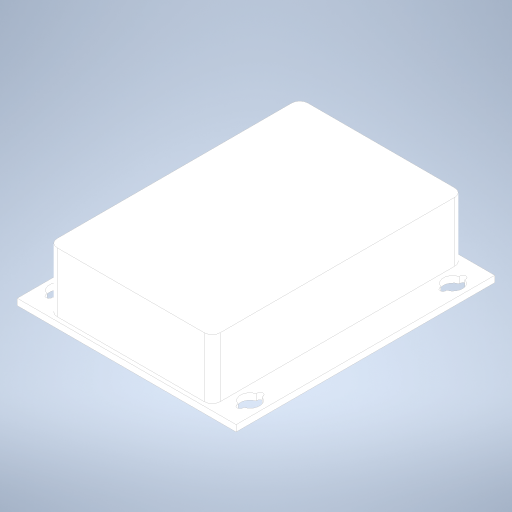
# Autodesk Inventor part: SUSTAINA-POWER-DISTRIBUTION-BOARD
Saved by Autodesk Inventor 2024.2 (Build 282272000, 272)
## iProperties
Created: 2024-01-24
Part Number: SUSTAINA-POWER-DISTRIBUTION-BOARD
Material: Acetal Resin, Black
Document SubType Name: Modeling
Designer: Masato Kubotera
Density: 1.425 g/cm^3
Appearance: Smooth - Black
Mass: 96.6275 g
Surface Area: 146.337 cm^2
Volume: 67.8088 cm^3
Author: Masato Kubotera
Autodesk Inventor part; units mm, degrees
ref_plane "YZ Plane" through (0, 0, 0) normal (1, 0, 0) x (0, 1, 0)
ref_plane "XZ Plane" through (0, 0, 0) normal (0, 1, 0) x (-1, 0, 0)
ref_plane "XY Plane" through (0, 0, 0) normal (0, 0, 1) x (1, 0, 0)
sketch "Sketch1" plane through (0, 0, 0) normal (0, 0, 1) x (1, 0, 0)
  line L0 (32.5, 27.5) -> (-32.5, 27.5)
  line L1 (-32.5, 27.5) -> (-32.5, -27.5)
  line L2 (-32.5, -27.5) -> (32.5, -27.5)
  line L3 (32.5, -27.5) -> (32.5, 27.5)
  line L4 (32.5, 27.5) -> (-32.5, -27.5) construction
  line L5 (-32.5, 27.5) -> (32.5, -27.5) construction
  line L6 (-25.5, 24) -> (25.5, 24) construction
  line L7 (25.5, 24) -> (25.5, -24) construction
  line L8 (25.5, -24) -> (-25.5, -24) construction
  line L9 (-25.5, -24) -> (-25.5, 24) construction
  line L10 (-25.5, 24) -> (25.5, -24) construction
  line L11 (25.5, 24) -> (-25.5, -24) construction
  line L12 (32.5, 0) -> (-32.5, 0) construction
  line L13 (0, 27.5) -> (0, -27.5) construction
  circle A0 centre (25.5, 24) radius 2.4
  circle A1 centre (-25.5, 24) radius 2.4
  circle A2 centre (25.5, -24) radius 2.4
  circle A3 centre (-25.5, -24) radius 2.4
  line L14 (25.5, 27.25) -> (25.5, 20.75) construction
  arc A4 (27.7895, 23.2801) -> (27.7895, 24.7199) centre (28, 24) ccw
  arc A5 (23.2105, 24.7199) -> (23.2105, 23.2801) centre (23, 24) ccw
  arc A6 (-27.7895, 24.7199) -> (-27.7895, 23.2801) centre (-28, 24) ccw
  arc A7 (-23.2105, 23.2801) -> (-23.2105, 24.7199) centre (-23, 24) ccw
  arc A8 (27.7895, -24.7199) -> (27.7895, -23.2801) centre (28, -24) ccw
  arc A9 (23.2105, -23.2801) -> (23.2105, -24.7199) centre (23, -24) ccw
  arc A10 (-27.7895, -23.2801) -> (-27.7895, -24.7199) centre (-28, -24) ccw
  arc A11 (-23.2105, -24.7199) -> (-23.2105, -23.2801) centre (-23, -24) ccw
  line L15 (31.5, 20.5) -> (-31.5, 20.5)
  line L16 (-31.5, 20.5) -> (-31.5, -20.5)
  line L17 (-31.5, -20.5) -> (31.5, -20.5)
  line L18 (31.5, -20.5) -> (31.5, 20.5)
  line L19 (31.5, 20.5) -> (-31.5, -20.5) construction
  line L20 (-31.5, 20.5) -> (31.5, -20.5) construction
  point P0 (0, 0)
  point P1 (28.75, 24)
  point P2 (22.25, 24)
  point P3 (28.75, -24)
  point P4 (23.2105, 23.2801)
  point P5 (23.2105, 24.7199)
  point P6 (-23.2105, 24.7199)
  point P7 (-23.2105, 23.2801)
  point P8 (-27.7895, 23.2801)
  point P9 (-27.7895, 24.7199)
  point P10 (-23.2105, -23.2801)
  point P11 (-23.2105, -24.7199)
  point P12 (-27.7895, -24.7199)
  point P13 (-27.7895, -23.2801)
  point P14 (27.7895, -23.2801)
  point P15 (27.7895, -24.7199)
  point P16 (23.2105, -24.7199)
  point P17 (23.2105, -23.2801)
  dimension "d0" = 65
  dimension "d1" = 55
  dimension "d19" = 4.8
  dimension "d30" = 6.5
  dimension "d33" = 48
  dimension "d34" = 51
  dimension "d35" = 6.5
  dimension "d36" = 1.5
  dimension "d37" = 7
  dimension "d38" = 1
  dimension "d39" = 41
  dimension "d40" = 63
  dimension "d41" = 14
  constraints: 42 end point, 25 symmetric about line, 20 point on circle, 12 centre point, 11 midpoint, 6 coincident, 6 parallel, 3 horizontal, 3 perpendicular, 1 point on line, 1 vertical, 11 other
  measures "d0" distance of L2.end L1.end
  measures "d1" distance of L1.end L0.end
  measures "d19" diameter of A0
  measures "d30" distance of L14.start L14.end
  measures "d33" distance of L8.end L6.start
  measures "d34" distance of L7.end L8.end
  measures "d35" distance of point (28.75, 24) point (22.25, 24)
  measures "d36" diameter of A4
  measures "d37" diameter of L0 L6
  measures "d38" distance between parallel lines of L3 L18
  measures "d39" distance of L15.end L16.end
  measures "d40" distance of L15.start L15.end
  measures "d41" diameter of L3 L7
extrude "Extrusion1" add sketch "Sketch1" along normal blind 1.6 contours L3 L2 L1 L0 | L18 L17 L16 L15
extrude "Extrusion2" add sketch "Sketch1" along normal blind 16.6 contours L18 L17 L16 L15
fillet "Fillet1" radius 2 4 edges at (31.5, -20.5, 9.1) (31.5, 20.5, 9.1) (-31.5, -20.5, 9.1) (-31.5, 20.5, 9.1)
body "Solid1"
